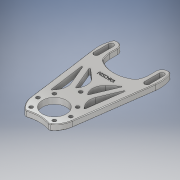
# Autodesk Inventor part: Motor Holder v3
Saved by Autodesk Inventor 2019.3 (Build 233278000, 278)
## iProperties
Created: 2019-03-01
Part Number: Motor Holder v3
Material: Aluminum 6061-AHC
Document SubType Name: Modeling
Designer: Petar
Density: 2.7 g/cm^3
Appearance: Aluminum - Dark
Mass: 26.5004 g
Surface Area: 70.5339 cm^2
Volume: 9.81495 cm^3
Author: Petar
Autodesk Inventor part; units mm, degrees
note: some values were not read from the file. Chosen so that the rebuilt part matches the saved one: direction of "Emboss1"; direction of "Emboss2".
ref_plane "YZ Plane" through (0, 0, 0) normal (1, 0, 0) x (0, 1, 0)
ref_plane "XZ Plane" through (0, 0, 0) normal (0, 1, 0) x (-1, 0, 0)
ref_plane "XY Plane" through (0, 0, 0) normal (0, 0, 1) x (1, 0, 0)
sketch "Sketch1" plane through (0, 0, 0) normal (0, 1, 0) x (-1, 0, 0)
  line L0 (0, 0) -> (0, 62.5) construction
  circle A0 centre (0, 62.5) radius 10
  line L1 (16, -6.25) -> (16, 0)
  line L2 (21.213203, 18.803327) -> (21.213203, -15.196673) construction
  line L3 (-21.213203, 18) -> (-21.213203, -16) construction
  circle A1 centre (21.213203, 3.5) radius 1.75 construction
  circle A2 centre (21.213203, -3.5) radius 1.75 construction
  circle A3 centre (-21.213203, 3.5) radius 1.75 construction
  circle A4 centre (-21.213203, -3.5) radius 1.75 construction
  line L4 (-16, -6.25) -> (-16, 0)
  line L5 (21.213203, 6.25) -> (21.213203, -6.25) construction
  line L6 (19.213203, 6.25) -> (19.213203, -6.25)
  line L7 (23.213203, -6.25) -> (23.213203, 6.25)
  arc A5 (23.213203, 6.25) -> (19.213203, 6.25) centre (21.213203, 6.25) ccw
  arc A6 (19.213203, -6.25) -> (23.213203, -6.25) centre (21.213203, -6.25) ccw
  line L8 (-19.213203, 6.25) -> (-19.213203, -6.25)
  line L9 (-23.213203, -6.25) -> (-23.213203, 6.25)
  arc A7 (-19.213203, 6.25) -> (-23.213203, 6.25) centre (-21.213203, 6.25) ccw
  arc A8 (-23.213203, -6.25) -> (-19.213203, -6.25) centre (-21.213203, -6.25) ccw
  arc A9 (14.049513, 52.066344) -> (17.337405, 64.88) centre (0, 62.5) ccw construction
  arc A10 (16, -6.25) -> (23.615648, -10.876635) centre (21.213203, -6.25) ccw
  arc A11 (-23.615648, -10.876635) -> (-16, -6.25) centre (-21.213203, -6.25) ccw
  line L10 (17.337405, 64.88) -> (25.75843, 3.536)
  line L11 (-17.337405, 64.88) -> (-25.75843, 3.536)
  circle A12 centre (0, 62.5) radius 13.75 construction
  circle A13 centre (9.722718, 72.222718) radius 1.5
  circle A14 centre (9.722718, 52.777282) radius 1.5
  line L12 (0, 62.5) -> (9.722718, 72.222718) construction
  line L13 (9.722718, 52.777282) -> (0, 62.5) construction
  circle A15 centre (-9.722718, 72.222718) radius 1.5
  circle A16 centre (-9.722718, 52.777282) radius 1.5
  circle A17 centre (13.75, 62.5) radius 1.5
  line L14 (13.75, 62.5) -> (0, 62.5) construction
  circle A18 centre (-13.75, 62.5) radius 1.5
  circle A19 centre (0, 40.5) radius 1.5
  line L15 (14.049513, 52.066344) -> (18.720045, 18.043279)
  arc A20 (17.337405, 64.88) -> (-17.337405, 64.88) centre (0, 62.5) ccw
  arc A21 (-17.337405, 64.88) -> (-14.049513, 52.066344) centre (0, 62.5) ccw construction
  line L16 (-14.049513, 52.066344) -> (-18.720045, 18.043279)
  line L17 (10, 76.861407) -> (0, 73.5) construction
  line L18 (0, 73.5) -> (-10, 76.861407) construction
  spline S0 degree 2 poles (10, 76.861407) (0, 73.5) (-10, 76.861407) knots 1 1 1 2 2 2
  line L19 (10, 76.861407) -> (-10, 76.861407) construction
  line L20 (18.720045, 18.043279) -> (-18.720045, 18.043279) construction
  line L21 (18.720045, 18.043279) -> (10.322856, 38.00336)
  line L22 (14.049513, 52.066344) -> (11.628469, 48.80627)
  arc A22 (11.628469, 48.80627) -> (10.322856, 38.00336) centre (20.442482, 42.260678) ccw
  line L23 (-18.720045, 18.043279) -> (-10.322856, 38.00336)
  line L24 (-14.049513, 52.066344) -> (-11.628469, 48.80627)
  arc A23 (-10.322856, 38.00336) -> (-11.628469, 48.80627) centre (-20.442482, 42.260678) ccw
  line L25 (14.380482, 18.043279) -> (5.123534, 40.047003)
  line L26 (14.380482, 18.043279) -> (5.876734, 25.327139)
  line L27 (5.123534, 40.047003) -> (4.341411, 38.993829)
  arc A24 (4.341411, 38.993829) -> (5.876734, 25.327139) centre (12.434727, 32.983452) ccw
  line L28 (-14.380482, 18.043279) -> (-5.123534, 40.047003)
  line L29 (-14.380482, 18.043279) -> (-5.876734, 25.327139)
  line L30 (-5.123534, 40.047003) -> (-4.341411, 38.993829)
  arc A25 (-5.876734, 25.327139) -> (-4.341411, 38.993829) centre (-12.434727, 32.983452) ccw
  arc A26 (23.615648, -10.876635) -> (26, 0) centre (0, 0) ccw
  arc A27 (-23.615648, -10.876635) -> (23.615648, -10.876635) centre (0, 0) ccw construction
  arc A28 (-12.306084, 22.903282) -> (-25.75843, 3.536) centre (0, 0) ccw construction
  line L31 (21.213203, -11.463203) -> (-21.213203, -11.463203) construction
  line L32 (-21.213203, 80) -> (25, 80) construction
  line L33 (0, 73.5) -> (0, 72.5) construction
  arc A29 (13.760985, 8.163043) -> (-13.760985, 8.163043) centre (0, -11.5) ccw
  line L34 (13.760985, 8.163043) -> (-13.760985, 8.163043) construction
  arc A30 (16, 0) -> (13.760985, 8.163043) centre (0, 0) ccw
  arc A31 (-13.760985, 8.163043) -> (-16, 0) centre (0, 0) ccw
  arc A32 (26, 0) -> (25.75843, 3.536) centre (0, 0) ccw
  arc A33 (-26, 0) -> (-23.615648, -10.876635) centre (0, 0) ccw
  arc A34 (-25.75843, 3.536) -> (-26, 0) centre (0, 0) ccw
  arc A35 (25.75843, 3.536) -> (-12.344609, 22.88254) centre (0, 0) ccw construction
  line L35 (16, 0) -> (-16, 0) construction
  point P0 (21.213203, 0)
  point P1 (0, 12.5)
  dimension "d1" = 20
  dimension "d0" = 62.5
  dimension "d3" = 3.5
  dimension "d4" = 3.5
  dimension "d5" = 7
  dimension "d7" = 43
  dimension "d9" = 3.5
  dimension "d11" = 32
  dimension "d15" = 4
  dimension "d24" = 3
  dimension "d25" = 3
  dimension "d27" = 45
  dimension "d29" = 3
  dimension "d30" = 3
  dimension "d31" = 22
  dimension "d50" = 20
  dimension "d53" = 26
  dimension "d75" = 91.4632
  dimension "d76" = 7.5
  dimension "d77" = 3.75
  dimension "d78" = 1
  dimension "d81" = 6.25
  dimension "d82" = 12.5
  dimension "d85" = 5
  dimension "d86" = 4
  dimension "d98" = 15
  dimension "d99" = 24
  constraints: 70 end point, 58 point on circle, 35 centre point, 26 symmetric about line, 19 tangent, 13 point on line, 7 coincident, 5 horizontal, 5 vertical, 3 parallel, 2 perpendicular, 1 collinear, 1 midpoint, 1 vertical alignment, 16 other
  measures "d0" distance of L0.start L0.end
  measures "d3" diameter of A1
  measures "d4" diameter of A2
  measures "d5" distance of A2.centre A1.centre
  measures "d7" distance of A2.centre A3.centre
  measures "d9" vertical distance of L0.start A1.centre
  measures "d11" distance between parallel lines of L4 L1
  measures "d15" distance between parallel lines of L6 L7
  measures "d24" diameter of A13
  measures "d25" diameter of A14
  measures "d27" angle of L0 L13
  measures "d29" diameter of A17
  measures "d30" diameter of A19
  measures "d31" distance of L0.end A19.centre
  measures "d50" distance of L17.start L18.end
  measures "d53" radius of A26
  measures "d75" distance between parallel lines of L31 L32
  measures "d78" distance of L33.start L33.end
  measures "d81" vertical distance of L5.start point (0, 12.5)
  measures "d82" distance of L5.end L5.start
  measures "d85" distance between parallel lines of L10 L15
  measures "d86" distance between parallel lines of L21 L25
  measures "d98" angle of L15 L21
  measures "d99" radius of A29
extrude "Extrusion3" add sketch "Sketch1" along normal blind 5 contours L1 A30 A29 A31 L4 A11 A33 A34 L11 A20 S0 L10 A32 A26 A10
thread "Thread1" size "M3x0.5" class "6H" standard "ANSI Metric M Profile" full length
thread "Thread2" size "M3x0.5" class "6H" standard "ANSI Metric M Profile" full length
thread "Thread3" size "M3x0.5" class "6H" standard "ANSI Metric M Profile" full length
thread "Thread4" size "M3x0.5" class "6H" standard "ANSI Metric M Profile" full length
thread "Thread5" size "M3x0.5" class "6H" standard "ANSI Metric M Profile" full length
thread "Thread6" size "M3x0.5" class "6H" standard "ANSI Metric M Profile" full length
thread "Thread7" size "M3x0.5" class "6H" standard "ANSI Metric M Profile" full length
sketch "Sketch3" plane through (0, 5, 0) normal (0, 1, 0) x (1, 0, 0)
  line L0 (-7.5, -16.5) -> (7.5, -16.5) construction
  line L1 (7.5, -16.5) -> (7.5, -21.5) construction
  line L2 (7.5, -21.5) -> (-7.5, -21.5) construction
  line L3 (-7.5, -21.5) -> (-7.5, -16.5) construction
  line L4 (0, 0.17633) -> (0, -59.82367) construction
  circle A0 centre (0, -62.5) radius 10
  arc A1 (-13.760985, -8.163043) -> (13.760985, -8.163043) centre (0, 11.5) ccw
  spline S0 degree 2 poles (-5.043979, -18.495705) (-5.043979, -18.660373) (-5.161305, -18.956775) (-5.266281, -19.059692) knots 0 0 0 1 2 2 2
  spline S1 degree 2 poles (-5.266281, -19.059692) (-5.398015, -19.189368) (-5.754109, -19.323161) (-6.025811, -19.323161) knots 0 0 0 1 2 2 2
  line L5 (-6.025811, -19.323161) -> (-6.311921, -19.323161)
  line L6 (-6.311921, -19.323161) -> (-6.311921, -20.27)
  line L7 (-6.311921, -20.27) -> (-6.64949, -20.27)
  line L8 (-6.64949, -20.27) -> (-6.64949, -17.73)
  line L9 (-6.64949, -17.73) -> (-6.011402, -17.73)
  spline S2 degree 2 poles (-6.011402, -17.73) (-5.784984, -17.73) (-5.467998, -17.8041) (-5.346556, -17.888493) knots 0 0 0 1 2 2 2
  spline S3 degree 2 poles (-5.346556, -17.888493) (-5.20453, -17.985235) (-5.043979, -18.283695) (-5.043979, -18.495705) knots 0 0 0 1 2 2 2
  spline S4 degree 2 poles (-5.395956, -18.505997) (-5.395956, -18.374263) (-5.486524, -18.180778) (-5.579149, -18.119028) knots 0 0 0 1 2 2 2
  spline S5 degree 2 poles (-5.579149, -18.119028) (-5.659425, -18.065511) (-5.873493, -18.022285) (-6.031986, -18.022285) knots 0 0 0 1 2 2 2
  line L10 (-6.031986, -18.022285) -> (-6.311921, -18.022285)
  line L11 (-6.311921, -18.022285) -> (-6.311921, -19.034992)
  line L12 (-6.311921, -19.034992) -> (-6.081386, -19.034992)
  spline S6 degree 2 poles (-6.081386, -19.034992) (-5.875551, -19.034992) (-5.622375, -18.969125) (-5.540041, -18.882674) knots 0 0 0 1 2 2 2
  spline S7 degree 2 poles (-5.540041, -18.882674) (-5.463882, -18.806515) (-5.395956, -18.627439) (-5.395956, -18.505997) knots 0 0 0 1 2 2 2
  line L13 (-3.837788, -20.27) -> (-4.821678, -20.27)
  line L14 (-4.821678, -20.27) -> (-4.821678, -20.010648)
  line L15 (-4.821678, -20.010648) -> (-4.498517, -20.010648)
  line L16 (-4.498517, -20.010648) -> (-4.498517, -17.989352)
  line L17 (-4.498517, -17.989352) -> (-4.821678, -17.989352)
  line L18 (-4.821678, -17.989352) -> (-4.821678, -17.73)
  line L19 (-4.821678, -17.73) -> (-3.837788, -17.73)
  line L20 (-3.837788, -17.73) -> (-3.837788, -17.989352)
  line L21 (-3.837788, -17.989352) -> (-4.160948, -17.989352)
  line L22 (-4.160948, -17.989352) -> (-4.160948, -20.010648)
  line L23 (-4.160948, -20.010648) -> (-3.837788, -20.010648)
  line L24 (-3.837788, -20.010648) -> (-3.837788, -20.27)
  spline S8 degree 2 poles (-2.711872, -20.315284) (-2.98769, -20.315284) (-3.37466, -20.200016) (-3.545502, -20.117682) knots 0 0 0 1 2 2 2
  line L25 (-3.545502, -20.117682) -> (-3.545502, -19.693663)
  line L26 (-3.545502, -19.693663) -> (-3.520802, -19.693663)
  spline S9 degree 2 poles (-3.520802, -19.693663) (-3.354076, -19.850097) (-2.932115, -20.022998) (-2.736572, -20.022998) knots 0 0 0 1 2 2 2
  spline S10 degree 2 poles (-2.736572, -20.022998) (-2.456637, -20.022998) (-2.170527, -19.790405) (-2.170527, -19.598979) knots 0 0 0 1 2 2 2
  spline S11 degree 2 poles (-2.170527, -19.598979) (-2.170527, -19.446661) (-2.320786, -19.257293) (-2.483395, -19.209951) knots 0 0 0 1 2 2 2
  spline S12 degree 2 poles (-2.483395, -19.209951) (-2.600721, -19.177018) (-2.796264, -19.131734) (-2.942407, -19.094684) knots 0 0 0 1 2 2 2
  spline S13 degree 2 poles (-2.942407, -19.094684) (-3.074141, -19.059692) (-3.282034, -18.954716) (-3.36231, -18.870324) knots 0 0 0 1 2 2 2
  spline S14 degree 2 poles (-3.36231, -18.870324) (-3.440527, -18.785932) (-3.526977, -18.559514) (-3.526977, -18.411313) knots 0 0 0 1 2 2 2
  spline S15 degree 2 poles (-3.526977, -18.411313) (-3.526977, -18.102561) (-3.045324, -17.684716) (-2.672763, -17.684716) knots 0 0 0 1 2 2 2
  spline S16 degree 2 poles (-2.672763, -17.684716) (-2.458695, -17.684716) (-2.079959, -17.769109) (-1.91735, -17.849384) knots 0 0 0 1 2 2 2
  line L27 (-1.91735, -17.849384) -> (-1.91735, -18.25282)
  line L28 (-1.91735, -18.25282) -> (-1.94205, -18.25282)
  spline S17 degree 2 poles (-1.94205, -18.25282) (-2.063493, -18.141669) (-2.442229, -17.977002) (-2.650122, -17.977002) knots 0 0 0 1 2 2 2
  spline S18 degree 2 poles (-2.650122, -17.977002) (-2.884773, -17.977002) (-3.175, -18.197245) (-3.175, -18.376321) knots 0 0 0 1 2 2 2
  spline S19 degree 2 poles (-3.175, -18.376321) (-3.175, -18.536872) (-3.004157, -18.728298) (-2.843606, -18.771524) knots 0 0 0 1 2 2 2
  spline S20 degree 2 poles (-2.843606, -18.771524) (-2.736572, -18.80034) (-2.425762, -18.874441) (-2.322844, -18.905316) knots 0 0 0 1 2 2 2
  spline S21 degree 2 poles (-2.322844, -18.905316) (-2.061434, -18.985592) (-1.818549, -19.308752) (-1.818549, -19.545462) knots 0 0 0 1 2 2 2
  spline S22 degree 2 poles (-1.818549, -19.545462) (-1.818549, -19.695721) (-1.939992, -19.98389) (-2.049084, -20.084749) knots 0 0 0 1 2 2 2
  spline S23 degree 2 poles (-2.049084, -20.084749) (-2.170527, -20.1959) (-2.479279, -20.315284) (-2.711872, -20.315284) knots 0 0 0 1 2 2 2
  spline S24 degree 2 poles (-0.482682, -20.315284) (-0.729684, -20.315284) (-1.147528, -20.148558) (-1.299846, -19.981832) knots 0 0 0 1 2 2 2
  spline S25 degree 2 poles (-1.299846, -19.981832) (-1.452164, -19.817164) (-1.61889, -19.323161) (-1.61889, -19.002058) knots 0 0 0 1 2 2 2
  spline S26 degree 2 poles (-1.61889, -19.002058) (-1.61889, -18.683015) (-1.45628, -18.209595) (-1.301904, -18.034635) knots 0 0 0 1 2 2 2
  spline S27 degree 2 poles (-1.301904, -18.034635) (-1.149587, -17.863793) (-0.733801, -17.684716) (-0.476507, -17.684716) knots 0 0 0 1 2 2 2
  spline S28 degree 2 poles (-0.476507, -17.684716) (-0.34889, -17.684716) (-0.12453, -17.721767) (-0.029846, -17.750583) knots 0 0 0 1 2 2 2
  spline S29 degree 2 poles (-0.029846, -17.750583) (0.052488, -17.777342) (0.223331, -17.853501) (0.307723, -17.898784) knots 0 0 0 1 2 2 2
  line L29 (0.307723, -17.898784) -> (0.307723, -18.306337)
  line L30 (0.307723, -18.306337) -> (0.280964, -18.306337)
  spline S30 degree 2 poles (0.280964, -18.306337) (0.235681, -18.26517) (0.095713, -18.149903) (-0.005146, -18.094327) knots 0 0 0 1 2 2 2
  spline S31 degree 2 poles (-0.005146, -18.094327) (-0.101888, -18.04081) (-0.330365, -17.972885) (-0.478566, -17.972885) knots 0 0 0 1 2 2 2
  spline S32 degree 2 poles (-0.478566, -17.972885) (-0.641175, -17.972885) (-0.931402, -18.106677) (-1.040494, -18.234295) knots 0 0 0 1 2 2 2
  spline S33 degree 2 poles (-1.040494, -18.234295) (-1.147528, -18.363971) (-1.266912, -18.757115) (-1.266912, -19.002058) knots 0 0 0 1 2 2 2
  spline S34 degree 2 poles (-1.266912, -19.002058) (-1.266912, -19.263468) (-1.141353, -19.640146) (-1.032261, -19.769822) knots 0 0 0 1 2 2 2
  spline S35 degree 2 poles (-1.032261, -19.769822) (-0.925227, -19.895381) (-0.639117, -20.022998) (-0.478566, -20.022998) knots 0 0 0 1 2 2 2
  spline S36 degree 2 poles (-0.478566, -20.022998) (-0.332423, -20.022998) (-0.083363, -19.950956) (0.013379, -19.897439) knots 0 0 0 1 2 2 2
  spline S37 degree 2 poles (0.013379, -19.897439) (0.106005, -19.843922) (0.243914, -19.732772) (0.283023, -19.693663) knots 0 0 0 1 2 2 2
  line L31 (0.283023, -19.693663) -> (0.307723, -19.693663)
  line L32 (0.307723, -19.693663) -> (0.307723, -20.097099)
  spline S38 degree 2 poles (0.307723, -20.097099) (0.223331, -20.136208) (0.07513, -20.20825) (-0.029846, -20.241183) knots 0 0 0 1 2 2 2
  spline S39 degree 2 poles (-0.029846, -20.241183) (-0.140997, -20.278233) (-0.330365, -20.315284) (-0.482682, -20.315284) knots 0 0 0 1 2 2 2
  line L33 (2.466929, -20.27) -> (2.12936, -20.27)
  line L34 (2.12936, -20.27) -> (2.12936, -19.026759)
  line L35 (2.12936, -19.026759) -> (0.960219, -19.026759)
  line L36 (0.960219, -19.026759) -> (0.960219, -20.27)
  line L37 (0.960219, -20.27) -> (0.62265, -20.27)
  line L38 (0.62265, -20.27) -> (0.62265, -17.73)
  line L39 (0.62265, -17.73) -> (0.960219, -17.73)
  line L40 (0.960219, -17.73) -> (0.960219, -18.72624)
  line L41 (0.960219, -18.72624) -> (2.12936, -18.72624)
  line L42 (2.12936, -18.72624) -> (2.12936, -17.73)
  line L43 (2.12936, -17.73) -> (2.466929, -17.73)
  line L44 (2.466929, -17.73) -> (2.466929, -20.27)
  line L45 (4.834028, -20.27) -> (4.3956, -20.27)
  line L46 (4.3956, -20.27) -> (3.467285, -19.088509)
  line L47 (3.467285, -19.088509) -> (3.319084, -19.255235)
  line L48 (3.319084, -19.255235) -> (3.319084, -20.27)
  line L49 (3.319084, -20.27) -> (2.981516, -20.27)
  line L50 (2.981516, -20.27) -> (2.981516, -17.73)
  line L51 (2.981516, -17.73) -> (3.319084, -17.73)
  line L52 (3.319084, -17.73) -> (3.319084, -18.897083)
  line L53 (3.319084, -18.897083) -> (4.360608, -17.73)
  line L54 (4.360608, -17.73) -> (4.772277, -17.73)
  line L55 (4.772277, -17.73) -> (3.720462, -18.864149)
  line L56 (3.720462, -18.864149) -> (4.834028, -20.27)
  line L57 (4.761986, -20.27) -> (5.618258, -17.73)
  line L58 (5.618258, -17.73) -> (6.034044, -17.73)
  line L59 (6.034044, -17.73) -> (6.890316, -20.27)
  line L60 (6.890316, -20.27) -> (6.534222, -20.27)
  line L61 (6.534222, -20.27) -> (6.303687, -19.55987)
  line L62 (6.303687, -19.55987) -> (5.334206, -19.55987)
  line L63 (5.334206, -19.55987) -> (5.103671, -20.27)
  line L64 (5.103671, -20.27) -> (4.761986, -20.27)
  line L65 (6.211062, -19.271702) -> (5.817918, -18.075802)
  line L66 (5.817918, -18.075802) -> (5.426832, -19.271702)
  line L67 (5.426832, -19.271702) -> (6.211062, -19.271702)
  dimension "d69" = 5
  dimension "d70" = 15
  dimension "d101" = 28
  constraints: 2 end point, 1 point on line, 1 vertical, 3 other
  measures "d69" distance between parallel lines of L0 L2
  measures "d70" distance between parallel lines of L3 L1
  measures "d101" distance from line of A1.centre L0
emboss "Emboss1" sketch "Sketch3" operation cut depth 0.2 direction (0, -1, 0) contours S0 S1 L5 L6 L7 L8 L9 S2 S3 | L13 L14 L15 L16 L17 L18 L19 L20 L21 L22 L23 L24 | S8 L25 L26 S9 S10 S11 S12 S13 S14 S15 S16 L27 L28 S17 S18 S19 S20 S21 S22 S23 | S24 S25 S26 S27 S28 S29 L29 L30 S30 S31 S32 S33 S34 S35 S36 S37 L31 L32 S38 S39 | L33 L34 L35 L36 L37 L38 L39 L40 L41 L42 L43 L44 | L45 L57 L56 | L56 L57 L58 L59 L60 L61 L62 L63 L64 | L45 L46 L47 L48 L49 L50 L51 L52 L53 L54 L55 L56 L57
sketch "Sketch4" plane through (0, 0, 0) normal (0, -1, 0) x (1, 0, 0)
  circle A0 centre (0, 40.5) radius 1.5
  line L0 (7.5, 16.5) -> (-7.5, 16.5) construction
  line L1 (-7.5, 16.5) -> (-7.5, 21.5) construction
  line L2 (-7.5, 21.5) -> (7.5, 21.5) construction
  line L3 (7.5, 21.5) -> (7.5, 16.5) construction
  arc A1 (-10, 76.861407) -> (-17.337405, 64.88) centre (0, 62.5) ccw
  arc A2 (13.760985, 8.163043) -> (-13.760985, 8.163043) centre (0, -11.5) ccw
  line L4 (0, 62.5) -> (0, 21.5) construction
  spline S0 degree 2 poles (5.043979, 18.495705) (5.043979, 18.660373) (5.161305, 18.956775) (5.266281, 19.059692) knots 0 0 0 1 2 2 2
  spline S1 degree 2 poles (5.266281, 19.059692) (5.398015, 19.189368) (5.754109, 19.323161) (6.025811, 19.323161) knots 0 0 0 1 2 2 2
  line L5 (6.025811, 19.323161) -> (6.311921, 19.323161)
  line L6 (6.311921, 19.323161) -> (6.311921, 20.27)
  line L7 (6.311921, 20.27) -> (6.64949, 20.27)
  line L8 (6.64949, 20.27) -> (6.64949, 17.73)
  line L9 (6.64949, 17.73) -> (6.011402, 17.73)
  spline S2 degree 2 poles (6.011402, 17.73) (5.784984, 17.73) (5.467998, 17.8041) (5.346556, 17.888493) knots 0 0 0 1 2 2 2
  spline S3 degree 2 poles (5.346556, 17.888493) (5.20453, 17.985235) (5.043979, 18.283695) (5.043979, 18.495705) knots 0 0 0 1 2 2 2
  spline S4 degree 2 poles (5.395956, 18.505997) (5.395956, 18.374263) (5.486524, 18.180778) (5.579149, 18.119028) knots 0 0 0 1 2 2 2
  spline S5 degree 2 poles (5.579149, 18.119028) (5.659425, 18.065511) (5.873493, 18.022285) (6.031986, 18.022285) knots 0 0 0 1 2 2 2
  line L10 (6.031986, 18.022285) -> (6.311921, 18.022285)
  line L11 (6.311921, 18.022285) -> (6.311921, 19.034992)
  line L12 (6.311921, 19.034992) -> (6.081386, 19.034992)
  spline S6 degree 2 poles (6.081386, 19.034992) (5.875551, 19.034992) (5.622375, 18.969125) (5.540041, 18.882674) knots 0 0 0 1 2 2 2
  spline S7 degree 2 poles (5.540041, 18.882674) (5.463882, 18.806515) (5.395956, 18.627439) (5.395956, 18.505997) knots 0 0 0 1 2 2 2
  line L13 (3.837788, 20.27) -> (4.821678, 20.27)
  line L14 (4.821678, 20.27) -> (4.821678, 20.010648)
  line L15 (4.821678, 20.010648) -> (4.498517, 20.010648)
  line L16 (4.498517, 20.010648) -> (4.498517, 17.989352)
  line L17 (4.498517, 17.989352) -> (4.821678, 17.989352)
  line L18 (4.821678, 17.989352) -> (4.821678, 17.73)
  line L19 (4.821678, 17.73) -> (3.837788, 17.73)
  line L20 (3.837788, 17.73) -> (3.837788, 17.989352)
  line L21 (3.837788, 17.989352) -> (4.160948, 17.989352)
  line L22 (4.160948, 17.989352) -> (4.160948, 20.010648)
  line L23 (4.160948, 20.010648) -> (3.837788, 20.010648)
  line L24 (3.837788, 20.010648) -> (3.837788, 20.27)
  spline S8 degree 2 poles (2.711872, 20.315284) (2.98769, 20.315284) (3.37466, 20.200016) (3.545502, 20.117682) knots 0 0 0 1 2 2 2
  line L25 (3.545502, 20.117682) -> (3.545502, 19.693663)
  line L26 (3.545502, 19.693663) -> (3.520802, 19.693663)
  spline S9 degree 2 poles (3.520802, 19.693663) (3.354076, 19.850097) (2.932115, 20.022998) (2.736572, 20.022998) knots 0 0 0 1 2 2 2
  spline S10 degree 2 poles (2.736572, 20.022998) (2.456637, 20.022998) (2.170527, 19.790405) (2.170527, 19.598979) knots 0 0 0 1 2 2 2
  spline S11 degree 2 poles (2.170527, 19.598979) (2.170527, 19.446661) (2.320786, 19.257293) (2.483395, 19.209951) knots 0 0 0 1 2 2 2
  spline S12 degree 2 poles (2.483395, 19.209951) (2.600721, 19.177018) (2.796264, 19.131734) (2.942407, 19.094684) knots 0 0 0 1 2 2 2
  spline S13 degree 2 poles (2.942407, 19.094684) (3.074141, 19.059692) (3.282034, 18.954716) (3.36231, 18.870324) knots 0 0 0 1 2 2 2
  spline S14 degree 2 poles (3.36231, 18.870324) (3.440527, 18.785932) (3.526977, 18.559514) (3.526977, 18.411313) knots 0 0 0 1 2 2 2
  spline S15 degree 2 poles (3.526977, 18.411313) (3.526977, 18.102561) (3.045324, 17.684716) (2.672763, 17.684716) knots 0 0 0 1 2 2 2
  spline S16 degree 2 poles (2.672763, 17.684716) (2.458695, 17.684716) (2.079959, 17.769109) (1.91735, 17.849384) knots 0 0 0 1 2 2 2
  line L27 (1.91735, 17.849384) -> (1.91735, 18.25282)
  line L28 (1.91735, 18.25282) -> (1.94205, 18.25282)
  spline S17 degree 2 poles (1.94205, 18.25282) (2.063493, 18.141669) (2.442229, 17.977002) (2.650122, 17.977002) knots 0 0 0 1 2 2 2
  spline S18 degree 2 poles (2.650122, 17.977002) (2.884773, 17.977002) (3.175, 18.197245) (3.175, 18.376321) knots 0 0 0 1 2 2 2
  spline S19 degree 2 poles (3.175, 18.376321) (3.175, 18.536872) (3.004157, 18.728298) (2.843606, 18.771524) knots 0 0 0 1 2 2 2
  spline S20 degree 2 poles (2.843606, 18.771524) (2.736572, 18.80034) (2.425762, 18.874441) (2.322844, 18.905316) knots 0 0 0 1 2 2 2
  spline S21 degree 2 poles (2.322844, 18.905316) (2.061434, 18.985592) (1.818549, 19.308752) (1.818549, 19.545462) knots 0 0 0 1 2 2 2
  spline S22 degree 2 poles (1.818549, 19.545462) (1.818549, 19.695721) (1.939992, 19.98389) (2.049084, 20.084749) knots 0 0 0 1 2 2 2
  spline S23 degree 2 poles (2.049084, 20.084749) (2.170527, 20.1959) (2.479279, 20.315284) (2.711872, 20.315284) knots 0 0 0 1 2 2 2
  spline S24 degree 2 poles (0.482682, 20.315284) (0.729684, 20.315284) (1.147528, 20.148558) (1.299846, 19.981832) knots 0 0 0 1 2 2 2
  spline S25 degree 2 poles (1.299846, 19.981832) (1.452164, 19.817164) (1.61889, 19.323161) (1.61889, 19.002058) knots 0 0 0 1 2 2 2
  spline S26 degree 2 poles (1.61889, 19.002058) (1.61889, 18.683015) (1.45628, 18.209595) (1.301904, 18.034635) knots 0 0 0 1 2 2 2
  spline S27 degree 2 poles (1.301904, 18.034635) (1.149587, 17.863793) (0.733801, 17.684716) (0.476507, 17.684716) knots 0 0 0 1 2 2 2
  spline S28 degree 2 poles (0.476507, 17.684716) (0.34889, 17.684716) (0.12453, 17.721767) (0.029846, 17.750583) knots 0 0 0 1 2 2 2
  spline S29 degree 2 poles (0.029846, 17.750583) (-0.052488, 17.777342) (-0.223331, 17.853501) (-0.307723, 17.898784) knots 0 0 0 1 2 2 2
  line L29 (-0.307723, 17.898784) -> (-0.307723, 18.306337)
  line L30 (-0.307723, 18.306337) -> (-0.280964, 18.306337)
  spline S30 degree 2 poles (-0.280964, 18.306337) (-0.235681, 18.26517) (-0.095713, 18.149903) (0.005146, 18.094327) knots 0 0 0 1 2 2 2
  spline S31 degree 2 poles (0.005146, 18.094327) (0.101888, 18.04081) (0.330365, 17.972885) (0.478566, 17.972885) knots 0 0 0 1 2 2 2
  spline S32 degree 2 poles (0.478566, 17.972885) (0.641175, 17.972885) (0.931402, 18.106677) (1.040494, 18.234295) knots 0 0 0 1 2 2 2
  spline S33 degree 2 poles (1.040494, 18.234295) (1.147528, 18.363971) (1.266912, 18.757115) (1.266912, 19.002058) knots 0 0 0 1 2 2 2
  spline S34 degree 2 poles (1.266912, 19.002058) (1.266912, 19.263468) (1.141353, 19.640146) (1.032261, 19.769822) knots 0 0 0 1 2 2 2
  spline S35 degree 2 poles (1.032261, 19.769822) (0.925227, 19.895381) (0.639117, 20.022998) (0.478566, 20.022998) knots 0 0 0 1 2 2 2
  spline S36 degree 2 poles (0.478566, 20.022998) (0.332423, 20.022998) (0.083363, 19.950956) (-0.013379, 19.897439) knots 0 0 0 1 2 2 2
  spline S37 degree 2 poles (-0.013379, 19.897439) (-0.106005, 19.843922) (-0.243914, 19.732772) (-0.283023, 19.693663) knots 0 0 0 1 2 2 2
  line L31 (-0.283023, 19.693663) -> (-0.307723, 19.693663)
  line L32 (-0.307723, 19.693663) -> (-0.307723, 20.097099)
  spline S38 degree 2 poles (-0.307723, 20.097099) (-0.223331, 20.136208) (-0.07513, 20.20825) (0.029846, 20.241183) knots 0 0 0 1 2 2 2
  spline S39 degree 2 poles (0.029846, 20.241183) (0.140997, 20.278233) (0.330365, 20.315284) (0.482682, 20.315284) knots 0 0 0 1 2 2 2
  line L33 (-2.466929, 20.27) -> (-2.12936, 20.27)
  line L34 (-2.12936, 20.27) -> (-2.12936, 19.026759)
  line L35 (-2.12936, 19.026759) -> (-0.960219, 19.026759)
  line L36 (-0.960219, 19.026759) -> (-0.960219, 20.27)
  line L37 (-0.960219, 20.27) -> (-0.62265, 20.27)
  line L38 (-0.62265, 20.27) -> (-0.62265, 17.73)
  line L39 (-0.62265, 17.73) -> (-0.960219, 17.73)
  line L40 (-0.960219, 17.73) -> (-0.960219, 18.72624)
  line L41 (-0.960219, 18.72624) -> (-2.12936, 18.72624)
  line L42 (-2.12936, 18.72624) -> (-2.12936, 17.73)
  line L43 (-2.12936, 17.73) -> (-2.466929, 17.73)
  line L44 (-2.466929, 17.73) -> (-2.466929, 20.27)
  line L45 (-4.834028, 20.27) -> (-4.3956, 20.27)
  line L46 (-4.3956, 20.27) -> (-3.467285, 19.088509)
  line L47 (-3.467285, 19.088509) -> (-3.319084, 19.255235)
  line L48 (-3.319084, 19.255235) -> (-3.319084, 20.27)
  line L49 (-3.319084, 20.27) -> (-2.981516, 20.27)
  line L50 (-2.981516, 20.27) -> (-2.981516, 17.73)
  line L51 (-2.981516, 17.73) -> (-3.319084, 17.73)
  line L52 (-3.319084, 17.73) -> (-3.319084, 18.897083)
  line L53 (-3.319084, 18.897083) -> (-4.360608, 17.73)
  line L54 (-4.360608, 17.73) -> (-4.772277, 17.73)
  line L55 (-4.772277, 17.73) -> (-3.720462, 18.864149)
  line L56 (-3.720462, 18.864149) -> (-4.834028, 20.27)
  line L57 (-4.761986, 20.27) -> (-5.618258, 17.73)
  line L58 (-5.618258, 17.73) -> (-6.034044, 17.73)
  line L59 (-6.034044, 17.73) -> (-6.890316, 20.27)
  line L60 (-6.890316, 20.27) -> (-6.534222, 20.27)
  line L61 (-6.534222, 20.27) -> (-6.303687, 19.55987)
  line L62 (-6.303687, 19.55987) -> (-5.334206, 19.55987)
  line L63 (-5.334206, 19.55987) -> (-5.103671, 20.27)
  line L64 (-5.103671, 20.27) -> (-4.761986, 20.27)
  line L65 (-6.211062, 19.271702) -> (-5.817918, 18.075802)
  line L66 (-5.817918, 18.075802) -> (-5.426832, 19.271702)
  line L67 (-5.426832, 19.271702) -> (-6.211062, 19.271702)
  dimension "d71" = 5
  dimension "d72" = 15
  dimension "d102" = 28
  constraints: 2 end point, 1 midpoint, 1 point on line, 2 other
  measures "d71" distance between parallel lines of L2 L0
  measures "d72" distance between parallel lines of L3 L1
  measures "d102" distance from line of L0 A2.centre
emboss "Emboss2" sketch "Sketch4" operation cut depth 0.2 direction (0, 1, 0) contours S0 S1 L5 L6 L7 L8 L9 S2 S3 | L13 L14 L15 L16 L17 L18 L19 L20 L21 L22 L23 L24 | S8 L25 L26 S9 S10 S11 S12 S13 S14 S15 S16 L27 L28 S17 S18 S19 S20 S21 S22 S23 | S24 S25 S26 S27 S28 S29 L29 L30 S30 S31 S32 S33 S34 S35 S36 S37 L31 L32 S38 S39 | L33 L34 L35 L36 L37 L38 L39 L40 L41 L42 L43 L44 | L45 L57 L56 | L56 L57 L58 L59 L60 L61 L62 L63 L64 | L45 L46 L47 L48 L49 L50 L51 L52 L53 L54 L55 L56 L57
fillet "Fillet3" radius 0.5 8 edges at (-18.72, 2.5, 18.0433) (-14.3805, 2.5, 18.0433) (-5.1235, 2.5, 40.047) (-14.0495, 2.5, 52.0663) (5.1235, 2.5, 40.047) (14.0495, 2.5, 52.0663) (18.72, 2.5, 18.0433) (14.3805, 2.5, 18.0433)
fillet "Fillet5" radius 2 6 edges at (-10, 2.5, 76.8614) (10, 2.5, 76.8614) (23.6156, 2.5, -10.8766) (-23.6156, 2.5, -10.8766) (-13.761, 2.5, 8.163) (13.761, 2.5, 8.163)
chamfer "Chamfer3" distance 0.5 angle 45 40 edges at (15.2013, 5, 71.17) (21.5479, 5, 34.208) (10.0052, 5, 76.6087) (0, 5, 75.1807) (-10.0052, 5, 76.6087) (-15.2013, 5, 71.17) (-21.5479, 5, 34.208) (-25.7753, 5, -3.4105) (-23.4392, 5, -10.8298) (-18.0833, 5, -10.419) (-16, 5, -3.125) (-15.4929, 5, 3.9962) (-13.7269, 5, 8.124) (0, 5, 12.5) (13.7269, 5, 8.124) (15.4929, 5, 3.9962) (16, 5, -3.125) (18.0833, 5, -10.419) (23.4392, 5, -10.8298) (25.7753, 5, -3.4105) (0, 0, 75.1807) (10.0052, 0, 76.6087) (15.2013, 0, 71.17) (21.5479, 0, 34.208) (-10.0052, 0, 76.6087) (-15.2013, 0, 71.17) (-21.5479, 0, 34.208) (-25.7753, 0, -3.4105) (-23.4392, 0, -10.8298) (-18.0833, 0, -10.419) (-16, 0, -3.125) (-15.4929, 0, 3.9962) (-13.7269, 0, 8.124) (0, 0, 12.5) (13.7269, 0, 8.124) (15.4929, 0, 3.9962) (16, 0, -3.125) (18.0833, 0, -10.419) (23.4392, 0, -10.8298) (25.7753, 0, -3.4105)
sketch "Center Lines" plane through (0, 5, 0) normal (0, 1, 0) x (1, 0, 0)
  arc A0 (-23.213203, -6.25) -> (-19.213203, -6.25) centre (-21.213203, -6.25) ccw construction
  line L0 (-23.213203, -6.25) -> (-23.213203, 6.25) construction
  arc A1 (-19.213203, 6.25) -> (-23.213203, 6.25) centre (-21.213203, 6.25) ccw construction
  line L1 (-19.213203, 6.25) -> (-19.213203, -6.25) construction
  line L2 (-21.213203, -6.25) -> (-21.213203, 6.25) construction
  line L3 (19.213203, -6.25) -> (19.213203, 6.25) construction
  arc A2 (19.213203, -6.25) -> (23.213203, -6.25) centre (21.213203, -6.25) ccw construction
  line L4 (23.213203, 6.25) -> (23.213203, -6.25) construction
  arc A3 (23.213203, 6.25) -> (19.213203, 6.25) centre (21.213203, 6.25) ccw construction
  line L5 (21.213203, -6.25) -> (21.213203, 6.25) construction
  constraints: 4 end point, 2 vertical
body "Solid3"
